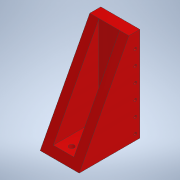
# Autodesk Inventor part: Slide Support
Saved by Autodesk Inventor 2022 (Build 260153000, 153)
## iProperties
Created: 2022-10-16
Part Number: Slide Support
Material: Generic
Document SubType Name: Modeling
Designer: matt
Density: 1 g/cm^3
Appearance: Default
Author: matt
Autodesk Inventor part; units mm, degrees
ref_plane "YZ Plane" through (0, 0, 0) normal (1, 0, 0) x (0, 1, 0)
ref_plane "XZ Plane" through (0, 0, 0) normal (0, 1, 0) x (-1, 0, 0)
ref_plane "XY Plane" through (0, 0, 0) normal (0, 0, 1) x (1, 0, 0)
sketch "Sketch1" plane through (0, 0, 0) normal (1, 0, 0) x (0, 1, 0)
  line L0 (0, 66) -> (0, 0)
  line L1 (-57.5, 0) -> (326.5, 0) construction
  line L2 (102.5, 12) -> (0, 12)
  circle A0 centre (6.5, 5) radius 1.5
  circle A1 centre (22.5, 5) radius 1.5
  circle A2 centre (38.5, 5) radius 1.5
  circle A3 centre (54.5, 5) radius 1.5
  circle A4 centre (70.5, 5) radius 1.5
  circle A5 centre (86.5, 5) radius 1.5
  line L3 (0, 0) -> (102.5, 0)
  line L4 (102.5, 0) -> (102.5, 12)
  line L5 (102.5, 66) -> (0, 66) construction
  line L6 (0, 66) -> (0, 0)
  line L7 (102.5, 12) -> (102.5, 66) construction
  line L8 (102.5, 12) -> (0, 66)
  line L9 (8, 0) -> (8, 61.7854)
  point P0 (8, 12)
  dimension "d0" = 12
  dimension "d1" = 3
  dimension "d2" = 5
  dimension "d3" = 6.5
  dimension "d6" = 16
  dimension "d11" = 16
  dimension "d12" = 66
  dimension "d19" = 8
  constraints: 20 end point, 6 centre point, 4 point on line, 3 parallel, 3 perpendicular, 2 horizontal, 1 coincident, 10 other
  measures "d0" distance between parallel lines of L2 L1
  measures "d1" diameter of A0
  measures "d2" distance from line of L1 A0.centre
  measures "d3" distance from line of L0 A0.centre
  measures "d6" distance of A0.centre A1.centre
  measures "d11" distance from line of L4 A5.centre
  measures "d12" distance between parallel lines of L5 L3
  measures "d19" distance between parallel lines of L0 L9
extrude "Extrusion1" add sketch "Sketch1" along normal blind 10 contours L8 L9 L2 L0 | A0 | L2 L9 L3 L0 | L8 L2 L9 | L2 L4 L3 L9 | A2 | A4
extrude "Extrusion2" add sketch "Sketch1" along normal blind 22.5 from surface at 10 contours L8 L9 L2 L0 | A0 | L2 L9 L3 L0 | L2 L4 L3 L9 | A2 | A4
extrude "Extrusion3" add sketch "Sketch1" along normal blind 10 from surface at 32.5 contours L8 L9 L2 L0 | A0 | L2 L9 L3 L0 | L8 L2 L9 | L2 L4 L3 L9 | A2 | A4
sketch "Sketch2" plane through (10, 8, 61.7854) normal (0, 1, 0) x (1, 0, 0)
  line L0 (22.5, 0) -> (22.5, 49.7854) projected
  line L1 (0, 49.7854) -> (22.5, 49.7854) projected
  line L2 (0, 0) -> (0, 49.7854) projected
  line L3 (0, 0) -> (22.5, 0) projected
  circle A0 centre (11.25, 40.8927) radius 2.8
  circle A1 centre (11.25, 8.8927) radius 2.8
  line L4 (0, 49.7854) -> (22.5, 49.7854) construction
  line L5 (11.25, 49.7854) -> (11.25, 0) construction
  line L6 (0, 0) -> (22.5, 0) construction
  point P0 (-10, 61.7854)
  dimension "d20" = 5.6
  dimension "d21" = 8.8927
  dimension "d22" = 49.7854
  dimension "d23" = 32
  constraints: 2 centre point, 2 end point, 2 midpoint
  measures "d20" diameter of A0
  measures "d21" distance from line of L1 A0.centre
  measures "d22" distance between parallel lines of L3 L1
  measures "d23" distance of A1.centre A0.centre
extrude "Extrusion4" cut sketch "Sketch2" against normal blind 22.5 contours A0 | A1
sketch "Sketch3" plane through (10, 8, 12) normal (0, 0, 1) x (1, 0, 0)
  line L0 (11.1125, 41.275) -> (11.1125, 12.7) construction
  line L1 (0.74, 41.275) -> (0.74, 12.7)
  line L2 (21.485, 12.7) -> (21.485, 41.275)
  arc A0 (21.485, 41.275) -> (0.74, 41.275) centre (11.1125, 41.275) ccw
  arc A1 (0.74, 12.7) -> (21.485, 12.7) centre (11.1125, 12.7) ccw
  point P0 (-10, -8)
  point P1 (11.1125, 26.9875)
  constraints: 8 end point, 4 point on circle, 4 tangent, 2 centre point, 1 midpoint, 1 parallel, 1 vertical
extrude "Extrusion5" cut sketch "Sketch3" against normal through all
equation "\"d21\" = -0.5 * d23 + 0.5 * d22"
body "Solid1"
